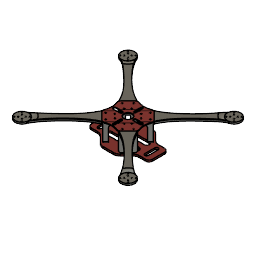
F450 Frame_GIT (Autodesk Fusion 360 design; units mm, degrees)
part number: 2026-06-03-11-10-49-567
Autodesk Fusion 360 part; units mm, degrees
sketch "Sketch1" plane through (0, 0, 0) normal (0, 0, 1) x (1, 0, 0)
  line L0 (-54, 54) -> (54, 54) construction
  line L1 (54, 54) -> (54, -54) construction
  line L2 (54, -54) -> (-54, -54) construction
  line L3 (-54, -54) -> (-54, 54) construction
  line L4 (-54, 54) -> (54, -54) construction
  line L5 (54, 54) -> (-54, -54) construction
  line L6 (-54, 24) -> (-24, 54)
  line L7 (24, 54) -> (54, 24)
  line L8 (54, -24) -> (24, -54)
  line L9 (-24, -54) -> (-54, -24)
  spline S0 degree 5 poles (-24, 54) (-23.04, 53.5449) (-21.12, 52.6745) (-18.24, 51.4881) (-14.4, 50.1486) (-9.6, 48.9056) (-4.8, 48.1327) (0, 47.868) (4.8, 48.1327) (9.6, 48.9056) (14.4, 50.1486) (18.24, 51.4881) (21.12, 52.6745) (23.04, 53.5449) (24, 54) knots 0 0 0 0 0 0 0.1 0.2 0.3 0.4 0.5 0.6 0.7 0.8 0.9 1 1 1 1 1 1
  spline S1 degree 5 poles (54, 24) (53.5449, 23.04) (52.6745, 21.12) (51.4881, 18.24) (50.1486, 14.4) (48.9056, 9.6) (48.1327, 4.8) (47.868, 0) (48.1327, -4.8) (48.9056, -9.6) (50.1486, -14.4) (51.4881, -18.24) (52.6745, -21.12) (53.5449, -23.04) (54, -24) knots 0 0 0 0 0 0 0.1 0.2 0.3 0.4 0.5 0.6 0.7 0.8 0.9 1 1 1 1 1 1
  spline S2 degree 5 poles (-24, -54) (-23.04, -53.5449) (-21.12, -52.6745) (-18.24, -51.4881) (-14.4, -50.1486) (-9.6, -48.9056) (-4.8, -48.1327) (0, -47.868) (4.8, -48.1327) (9.6, -48.9056) (14.4, -50.1486) (18.24, -51.4881) (21.12, -52.6745) (23.04, -53.5449) (24, -54) knots 0 0 0 0 0 0 0.1 0.2 0.3 0.4 0.5 0.6 0.7 0.8 0.9 1 1 1 1 1 1
  spline S3 degree 5 poles (-54, 24) (-53.5449, 23.04) (-52.6745, 21.12) (-51.4881, 18.24) (-50.1486, 14.4) (-48.9056, 9.6) (-48.1327, 4.8) (-47.868, 0) (-48.1327, -4.8) (-48.9056, -9.6) (-50.1486, -14.4) (-51.4881, -18.24) (-52.6745, -21.12) (-53.5449, -23.04) (-54, -24) knots 0 0 0 0 0 0 0.1 0.2 0.3 0.4 0.5 0.6 0.7 0.8 0.9 1 1 1 1 1 1
  circle A0 centre (-41.8284, 24.8579) radius 1.6
  circle A1 centre (-25.1436, 13.8299) radius 1.6
  circle A2 centre (-24.8579, 41.8284) radius 1.6
  circle A3 centre (-13.8299, 25.1436) radius 1.6
  line L10 (110, 0) -> (-135, 0) construction
  circle A4 centre (-13.8299, -25.1436) radius 1.6
  circle A5 centre (-25.1436, -13.8299) radius 1.6
  circle A6 centre (-41.8284, -24.8579) radius 1.6
  circle A7 centre (-24.8579, -41.8284) radius 1.6
  line L11 (0, 80) -> (0, -85.6972) construction
  circle A8 centre (41.8284, 24.8579) radius 1.6
  circle A9 centre (24.8579, 41.8284) radius 1.6
  circle A10 centre (13.8299, 25.1436) radius 1.6
  circle A11 centre (25.1436, 13.8299) radius 1.6
  circle A12 centre (25.1436, -13.8299) radius 1.6
  circle A13 centre (13.8299, -25.1436) radius 1.6
  circle A14 centre (24.8579, -41.8284) radius 1.6
  circle A15 centre (41.8284, -24.8579) radius 1.6
  point P0 (0, 48)
  point P1 (48, 0)
  point P2 (0, -48)
  point P3 (-48, 0)
  dimension "d1" = 108
  dimension "d2" = 108
  dimension "d3" = 30
  dimension "d4" = 30
  dimension "d5" = 30
  dimension "d6" = 45
  dimension "d7" = 30
  dimension "d8" = 45
  dimension "d9" = 6
  dimension "d10" = 6
  dimension "d11" = 6
  dimension "d12" = 6
  dimension "d13" = 3.2
  dimension "d14" = 3.2
  dimension "d15" = 8
  dimension "d16" = 12
  dimension "d17" = 8
  dimension "d18" = 20
  constraint horizontal L0
  constraint perpendicular L0 L1
  constraint parallel L0 L2
  constraint parallel L1 L3
  constraint coincident L4 origin
  constraint coincident L5 origin
  constraint coincident L3 L6.start
  constraint coincident L0 L6.end
  constraint coincident L0 L7.start
  constraint coincident L1 L7.end
  constraint coincident L1 L8.start
  constraint coincident L2 L8.end
  constraint perpendicular L4 L8
  constraint coincident L2 L9.start
  constraint coincident L3 L9.end
  constraint perpendicular L5 L9
  constraint symmetric L4 A0 A2
  constraint symmetric L4 A1 A3
  constraint horizontal L10
  constraint symmetric A0 L10 A6
  constraint symmetric A1 L10 A5
  constraint symmetric A2 L10 A7
  constraint symmetric A3 L10 A4
  constraint perpendicular L0 L11
  constraint symmetric A0 L11 A8
  constraint symmetric A1 L11 A11
  constraint symmetric A2 L11 A9
  constraint symmetric A3 L11 A10
  constraint symmetric A4 L11 A13
  constraint symmetric A5 L11 A12
  constraint symmetric A6 L11 A15
  constraint symmetric A7 L11 A14
  measures "d1" distance of L0.end L1.end
  measures "d2" distance of L0.start L0.end
  measures "d3" distance of L2.end L9.start
  measures "d4" distance of L1.end L8.end
  measures "d5" distance of L0.end L7.end
  measures "d6" angle of L0 L7
  measures "d7" distance of L0.start L6.end
  measures "d8" angle of L0 L6
  measures "d9" distance of L0 P0
  measures "d10" distance of L1 P1
  measures "d11" distance of L2 P2
  measures "d12" distance of L3 P3
  measures "d13" diameter of A0
  measures "d14" diameter of A1
  measures "d15" distance of L6 A0.centre
  measures "d16" distance of L4 A0.centre
  measures "d17" distance of L4 A1.centre
  measures "d18" distance of A0.centre A1.centre
extrude "Extrude1" add sketch "Sketch1" along normal blind 2 makes body 1
fillet "Fillet1" radius 10 8 edges at (-54, -24, 1) (-24, -54, 1) (24, -54, 1) (54, -24, 1) (-24, 54, 1) (-54, 24, 1) (24, 54, 1) (54, 24, 1) on bodies 1
sketch "Sketch2" plane through (0, 0, 2) normal (0, 0, 1) x (-1, 0, 0)
  spline S0 degree 3 poles (-49.2413, -28.7587) (-50.1621, -27.8379) (-50.8942, -26.7461) (-51.8987, -24.3434) (-52.1615, -23.0554) (-52.178, -20.5388) (-51.9647, -19.3329) (-51.5405, -18.1949) knots 0 0 0 0 0.390644 0.390644 0.781289 0.781289 1.145638 1.145638 1.145638 1.145638
  line L0 (-49.2413, -28.7587) -> (-28.7587, -49.2413)
  spline S1 degree 3 poles (-18.1949, -51.5405) (-19.4151, -51.9953) (-20.7124, -52.2074) (-23.3153, -52.1224) (-24.596, -51.8262) (-26.8918, -50.7953) (-27.8999, -50.1001) (-28.7587, -49.2413) knots 0 0 0 0 0.390644 0.390644 0.781289 0.781289 1.145638 1.145638 1.145638 1.145638
  spline S2 degree 5 poles (-18.1949, -51.5405) (-17.4359, -51.2576) (-15.717, -50.6459) (-13.038, -49.7969) (-9.399, -48.8733) (-4.8, -48.1327) (0, -47.868) (4.8, -48.1327) (9.399, -48.8733) (13.038, -49.7969) (15.717, -50.6459) (17.4359, -51.2576) (18.1949, -51.5405) knots -0.879061 -0.879061 -0.879061 -0.879061 -0.879061 -0.879061 -0.8 -0.7 -0.6 -0.5 -0.4 -0.3 -0.2 -0.120939 -0.120939 -0.120939 -0.120939 -0.120939 -0.120939
  spline S3 degree 3 poles (28.7587, -49.2413) (27.8379, -50.1621) (26.7461, -50.8942) (24.3434, -51.8987) (23.0554, -52.1615) (20.5388, -52.178) (19.3329, -51.9647) (18.1949, -51.5405) knots 0 0 0 0 0.390644 0.390644 0.781289 0.781289 1.145638 1.145638 1.145638 1.145638
  line L1 (28.7587, -49.2413) -> (49.2413, -28.7587)
  spline S4 degree 3 poles (51.5405, -18.1949) (51.9953, -19.4151) (52.2074, -20.7124) (52.1224, -23.3153) (51.8262, -24.596) (50.7953, -26.8918) (50.1001, -27.8999) (49.2413, -28.7587) knots 0 0 0 0 0.390644 0.390644 0.781289 0.781289 1.145638 1.145638 1.145638 1.145638
  spline S5 degree 5 poles (51.5405, -18.1949) (51.2576, -17.4359) (50.6459, -15.717) (49.7969, -13.038) (48.8733, -9.399) (48.1327, -4.8) (47.868, 0) (48.1327, 4.8) (48.8733, 9.399) (49.7969, 13.038) (50.6459, 15.717) (51.2576, 17.4359) (51.5405, 18.1949) knots 0.120939 0.120939 0.120939 0.120939 0.120939 0.120939 0.2 0.3 0.4 0.5 0.6 0.7 0.8 0.879061 0.879061 0.879061 0.879061 0.879061 0.879061
  spline S6 degree 3 poles (49.2413, 28.7587) (50.1621, 27.8379) (50.8942, 26.7461) (51.8987, 24.3434) (52.1615, 23.0554) (52.178, 20.5388) (51.9647, 19.3329) (51.5405, 18.1949) knots 0 0 0 0 0.390644 0.390644 0.781289 0.781289 1.145638 1.145638 1.145638 1.145638
  line L2 (49.2413, 28.7587) -> (28.7587, 49.2413)
  spline S7 degree 3 poles (18.1949, 51.5405) (19.4151, 51.9953) (20.7124, 52.2074) (23.3153, 52.1224) (24.596, 51.8262) (26.8918, 50.7953) (27.8999, 50.1001) (28.7587, 49.2413) knots 0 0 0 0 0.390644 0.390644 0.781289 0.781289 1.145638 1.145638 1.145638 1.145638
  spline S8 degree 5 poles (18.1949, 51.5405) (17.4359, 51.2576) (15.717, 50.6459) (13.038, 49.7969) (9.399, 48.8733) (4.8, 48.1327) (0, 47.868) (-4.8, 48.1327) (-9.399, 48.8733) (-13.038, 49.7969) (-15.717, 50.6459) (-17.4359, 51.2576) (-18.1949, 51.5405) knots 0.120939 0.120939 0.120939 0.120939 0.120939 0.120939 0.2 0.3 0.4 0.5 0.6 0.7 0.8 0.879061 0.879061 0.879061 0.879061 0.879061 0.879061
  spline S9 degree 3 poles (-28.7587, 49.2413) (-27.8379, 50.1621) (-26.7461, 50.8942) (-24.3434, 51.8987) (-23.0554, 52.1615) (-20.5388, 52.178) (-19.3329, 51.9647) (-18.1949, 51.5405) knots 0 0 0 0 0.390644 0.390644 0.781289 0.781289 1.145638 1.145638 1.145638 1.145638
  line L3 (-28.7587, 49.2413) -> (-49.2413, 28.7587)
  spline S10 degree 3 poles (-51.5405, 18.1949) (-51.9953, 19.4151) (-52.2074, 20.7124) (-52.1224, 23.3153) (-51.8262, 24.596) (-50.7953, 26.8918) (-50.1001, 27.8999) (-49.2413, 28.7587) knots 0 0 0 0 0.390644 0.390644 0.781289 0.781289 1.145638 1.145638 1.145638 1.145638
  spline S11 degree 5 poles (-51.5405, 18.1949) (-51.2576, 17.4359) (-50.6459, 15.717) (-49.7969, 13.038) (-48.8733, 9.399) (-48.1327, 4.8) (-47.868, 0) (-48.1327, -4.8) (-48.8733, -9.399) (-49.7969, -13.038) (-50.6459, -15.717) (-51.2576, -17.4359) (-51.5405, -18.1949) knots -0.879061 -0.879061 -0.879061 -0.879061 -0.879061 -0.879061 -0.8 -0.7 -0.6 -0.5 -0.4 -0.3 -0.2 -0.120939 -0.120939 -0.120939 -0.120939 -0.120939 -0.120939
  circle A0 centre (-24.8579, -41.8284) radius 1.6
  circle A1 centre (24.8579, -41.8284) radius 1.6
  circle A2 centre (-13.8299, -25.1436) radius 1.6
  circle A3 centre (25.1436, -13.8299) radius 1.6
  circle A4 centre (-13.8299, 25.1436) radius 1.6
  circle A5 centre (24.8579, 41.8284) radius 1.6
  circle A6 centre (41.8284, 24.8579) radius 1.6
  circle A7 centre (13.8299, -25.1436) radius 1.6
  circle A8 centre (-41.8284, -24.8579) radius 1.6
  circle A9 centre (41.8284, -24.8579) radius 1.6
  circle A10 centre (-41.8284, 24.8579) radius 1.6
  circle A11 centre (-24.8579, 41.8284) radius 1.6
  circle A12 centre (-25.1436, -13.8299) radius 1.6
  circle A13 centre (-25.1436, 13.8299) radius 1.6
  circle A14 centre (13.8299, 25.1436) radius 1.6
  circle A15 centre (25.1436, 13.8299) radius 1.6
  circle A16 centre (0, 0) radius 12.5
  line L4 (3, -42) -> (3, -20)
  arc A17 (3, -20) -> (-3, -20) centre (0, -20) ccw
  line L5 (-3, -20) -> (-3, -42)
  arc A18 (-3, -42) -> (3, -42) centre (0, -42) ccw
  line L6 (0, -42) -> (0, -20) construction
  line L7 (-20, 4) -> (-40, 4)
  arc A19 (-40, 4) -> (-40, -4) centre (-40, 0) ccw
  line L8 (-40, -4) -> (-20, -4)
  arc A20 (-20, -4) -> (-20, 4) centre (-20, 0) ccw
  line L9 (-20, 0) -> (-40, 0) construction
  line L10 (-77.8428, 0) -> (72.1572, 0) construction
  line L11 (0, -80) -> (0, 70) construction
  line L12 (40, -4) -> (20, -4)
  arc A21 (40, -4) -> (40, 4) centre (40, 0) ccw
  line L13 (20, 4) -> (40, 4)
  arc A22 (20, 4) -> (20, -4) centre (20, 0) ccw
  line L14 (-3, 20) -> (-3, 42)
  line L15 (3, 42) -> (3, 20)
  arc A23 (-3, 20) -> (3, 20) centre (0, 20) ccw
  arc A24 (3, 42) -> (-3, 42) centre (0, 42) ccw
  dimension "d23" = 25
  dimension "d24" = 6
  dimension "d25" = 8
  dimension "d26" = 20
  dimension "d27" = 150
  dimension "d28" = 150
  dimension "d29" = 20
  dimension "d30" = 20
  dimension "d31" = 22
  constraint coincident A16.centre origin
  constraint tangent L4 A17
  constraint tangent A17 L5
  constraint parallel L4 L5
  constraint tangent L5 A18
  constraint tangent L4 A18
  constraint vertical L6
  constraint tangent L7 A19
  constraint tangent A19 L8
  constraint parallel L7 L8
  constraint tangent L8 A20
  constraint tangent L7 A20
  constraint perpendicular L5 L9
  constraint horizontal L10
  constraint perpendicular L10 L11
  constraint collinear L9 L10
  constraint collinear L6 L11
  constraint symmetric L7.start L11 L13.start
  constraint symmetric L7.end L11 A21.end
  constraint symmetric A19.end L11 L12.start
  constraint symmetric L8.end L11 L12.end
  constraint symmetric A19 L11 A21
  constraint symmetric A20 L11 A22
  constraint symmetric L4.start L10 L15.start
  constraint symmetric L4.end L10 L15.end
  constraint symmetric A17.end L10 L14.start
  constraint symmetric L5.end L10 L14.end
  constraint symmetric A17 L10 A23
  constraint symmetric A18 L10 A24
  measures "d23" diameter of A16
  measures "d24" diameter of A17
  measures "d25" diameter of A19
  measures "d26" distance of A16.centre A20.centre
  measures "d27" distance of L10.start L10.end
  measures "d28" distance of L11.start L11.end
  measures "d29" distance of L7.start L7.end
  measures "d30" distance of A16.centre A17.centre
  measures "d31" distance of A17.end L5.end
extrude "Extrude2" cut sketch "Sketch2" against normal blind 2 contours A16 | L4 A17 L5 A18 | L7 A19 L8 A20 | L12 A21 L13 A22 | L14 L15 A23 A24 bodies 1
sketch "Sketch3" plane through (0, 0, 0) normal (0, 0, 1) x (1, 0, 0)
  line L0 (-65, 0) -> (70, 0) construction
  line L1 (0, -60) -> (0, 58.4085) construction
  line L2 (0, 0) -> (-176.7767, -176.7767) construction
  line L3 (-53.1421, -24.8579) -> (-24.8579, -53.1421)
  line L4 (-24.8579, -53.1421) -> (-6.4731, -34.7574)
  line L5 (-6.4731, -27.6863) -> (-27.6863, -6.4731)
  line L6 (-34.7574, -6.4731) -> (-53.1421, -24.8579)
  line L7 (-28.7587, -49.2413) -> (-49.2413, -28.7587)
  line L8 (-53.1421, -24.8579) -> (-171.9361, -143.6518) construction
  arc A0 (-27.6863, -6.4731) -> (-34.7574, -6.4731) centre (-31.2218, -10.0086) ccw
  arc A1 (-6.4731, -34.7574) -> (-6.4731, -27.6863) centre (-10.0086, -31.2218) ccw
  spline S0 degree 5 poles (-161.6105, -138.0992) (-160.6934, -137.7884) (-158.862, -137.1008) (-156.1235, -135.872) (-152.4419, -133.8154) (-147.5291, -130.4225) (-142.0023, -126.0691) (-135.6062, -120.6511) (-128.2424, -114.1593) (-120.0269, -106.7101) (-111.217, -98.5051) (-102.1675, -89.8068) (-93.2782, -80.9105) (-84.9455, -72.1182) (-77.5142, -63.7134) (-71.2254, -55.934) (-66.1683, -48.9471) (-62.2148, -42.8159) (-59.1194, -37.5347) (-56.6405, -33.0703) (-54.6445, -29.3984) (-53.5182, -27.1156) (-53.1237, -25.8179) (-53.0967, -25.1457) (-53.1421, -24.8579) knots 0 0 0 0 0 0 0.05 0.1 0.15 0.2 0.25 0.3 0.35 0.4 0.45 0.5 0.55 0.6 0.65 0.7 0.75 0.8 0.85 0.9 0.95 1 1 1 1 1 1
  line L9 (-51.7629, -33.5887) -> (-54.5214, -16.127)
  arc A2 (-162.4784, -138.3503) -> (-138.4805, -162.9894) centre (-157.7939, -157.7939) ccw
  spline S1 degree 5 poles (-137.3068, -160.2918) (-136.8023, -159.4836) (-135.7882, -157.8486) (-134.2519, -155.3405) (-132.1225, -151.8441) (-129.0449, -146.9999) (-125.2177, -141.4333) (-120.3455, -134.9473) (-114.2866, -127.4998) (-107.0974, -119.239) (-98.9687, -110.4365) (-90.1915, -101.4469) (-81.1134, -92.6595) (-72.101, -84.4542) (-63.5011, -77.1557) (-55.6013, -70.9864) (-48.5918, -66.0203) (-42.5198, -62.1251) (-37.3411, -59.0626) (-32.978, -56.603) (-29.3709, -54.6233) (-27.1046, -53.5111) (-25.8125, -53.123) (-25.1439, -53.0969) (-24.8579, -53.1421) knots 0 0 0 0 0 0 0.05 0.1 0.15 0.2 0.25 0.3 0.35 0.4 0.45 0.5 0.55 0.6 0.65 0.7 0.75 0.8 0.85 0.9 0.95 1 1 1 1 1 1
  line L10 (-33.5887, -51.7629) -> (-16.127, -54.5214)
  arc A3 (-162.4784, -138.3503) -> (-161.6105, -138.0992) centre (-164.8207, -128.6285) ccw
  arc A4 (-137.3068, -160.2918) -> (-138.4805, -162.9894) centre (-128.8238, -165.5871) ccw
  circle A5 centre (-169.3551, -169.3551) radius 1.6
  circle A6 centre (-163.3447, -163.3447) radius 1.6
  circle A7 centre (-152.2432, -163.3447) radius 1.6
  circle A8 centre (-146.2328, -169.3551) radius 1.6
  circle A9 centre (-152.2432, -152.2432) radius 1.6
  circle A10 centre (-146.2328, -146.2328) radius 1.6
  circle A11 centre (-163.3447, -152.2432) radius 1.6
  circle A12 centre (-169.3551, -146.2328) radius 1.6
  circle A13 centre (-41.8284, -24.8579) radius 1.6
  circle A14 centre (-25.1436, -13.8299) radius 1.6
  circle A15 centre (-13.8299, -25.1436) radius 1.6
  circle A16 centre (-24.8579, -41.8284) radius 1.6
  circle A17 centre (-41.8284, -24.8579) radius 2.5
  circle A18 centre (-24.8579, -41.8284) radius 2.5
  circle A19 centre (-13.8299, -25.1436) radius 2.5
  circle A20 centre (-25.1436, -13.8299) radius 2.5
  point P0 (-31.2218, -2.9376)
  point P1 (-137.4081, -122.1384)
  point P2 (-70.9005, -55.3064)
  point P3 (-55, -30)
  point P4 (-122.1384, -137.4081)
  point P5 (-55.3064, -70.9005)
  point P6 (-30, -55)
  dimension "d34" = 250
  dimension "d35" = 45
  dimension "d37" = 40
  dimension "d38" = 31
  dimension "d39" = 20
  dimension "d40" = 168
  dimension "d41" = 5
  dimension "d42" = 40
  dimension "d43" = 10
  dimension "d44" = 3.2
  dimension "d45" = 3.2
  dimension "d46" = 16.35
  dimension "d47" = 7.85
  dimension "d49" = 360
  dimension "d50" = 5
  dimension "d51" = 5
  dimension "d52" = 5
  dimension "d53" = 5
  constraint horizontal L0
  constraint perpendicular L0 L1
  constraint coincident L2.start origin
  constraint perpendicular L3 L4
  constraint parallel L3 L5
  constraint parallel L4 L6
  constraint perpendicular L2 L3
  constraint collinear L3 L7
  constraint parallel L2 L8
  constraint coincident P0 L5
  constraint coincident P0 L6
  constraint tangent L5 A0
  constraint tangent L6 A0
  constraint tangent L4 A1
  constraint tangent L5 A1
  constraint equal A0 A1
  constraint coincident L8.end A2
  constraint coincident L2 A2.centre
  constraint symmetric L2 L3.start L3.end
  constraint symmetric L2 P1 P4
  constraint symmetric L2 P2 P5
  constraint symmetric L2 P3 P6
  constraint midpoint L3.start L9
  constraint midpoint L3.end L10
  constraint tangent S0 A3
  constraint tangent A2 A3
  constraint tangent A2 A4
  constraint tangent S1 A4
  constraint equal A3 A4
  constraint coincident L2 A5.centre
  constraint coincident L2 A6.centre
  constraint concentric A13 A17
  constraint concentric A16 A18
  constraint concentric A15 A19
  constraint concentric A14 A20
  measures "d34" distance of L2.start L2.end
  measures "d35" angle of L1 L2
  measures "d37" distance of L3.start L3.end
  measures "d38" distance of L3.start P0
  measures "d39" distance of L2 L4
  measures "d40" distance of L3.start L8.end
  measures "d41" radius of A0
  measures "d42" diameter of A2
  measures "d43" radius of A3
  measures "d44" diameter of A5
  measures "d45" diameter of A6
  measures "d46" distance of A2.centre A5.centre
  measures "d47" distance of A2.centre A6.centre
  measures "d50" diameter of A17
  measures "d51" diameter of A18
  measures "d52" diameter of A19
  measures "d53" diameter of A20
extrude "Extrude3" add sketch "Sketch3" against normal blind 5 separate body contours L3 L4 L5 L6 L7 A0 A1 | L3 L7 S0 A2 S1 A3 A4 makes body 2
sketch "Sketch4" plane through (0, 0, -5) normal (0, 0, -1) x (1, 0, 0)
  circle A0 centre (-152.2432, 152.2432) radius 1.6
  circle A1 centre (-146.2328, 146.2328) radius 1.6
  line L0 (-6.4731, 34.7574) -> (-24.8579, 53.1421)
  spline S0 degree 5 poles (-24.8579, 53.1421) (-25.1439, 53.0969) (-25.8125, 53.123) (-27.1046, 53.5111) (-29.3709, 54.6233) (-32.978, 56.603) (-37.3411, 59.0626) (-42.5198, 62.1251) (-48.5918, 66.0203) (-55.6013, 70.9864) (-63.5011, 77.1557) (-72.101, 84.4542) (-81.1134, 92.6595) (-90.1915, 101.4469) (-98.9687, 110.4365) (-107.0974, 119.239) (-114.2866, 127.4998) (-120.3455, 134.9473) (-125.2177, 141.4333) (-129.0449, 146.9999) (-132.1225, 151.8441) (-134.2519, 155.3405) (-135.7882, 157.8486) (-136.8023, 159.4836) (-137.3068, 160.2918) knots -1 -1 -1 -1 -1 -1 -0.95 -0.9 -0.85 -0.8 -0.75 -0.7 -0.65 -0.6 -0.55 -0.5 -0.45 -0.4 -0.35 -0.3 -0.25 -0.2 -0.15 -0.1 -0.05 0 0 0 0 0 0
  arc A2 (-138.4805, 162.9894) -> (-137.3068, 160.2918) centre (-128.8238, 165.5871) ccw
  arc A3 (-138.4805, 162.9894) -> (-162.4784, 138.3503) centre (-157.7939, 157.7939) ccw
  arc A4 (-161.6105, 138.0992) -> (-162.4784, 138.3503) centre (-164.8207, 128.6285) ccw
  spline S1 degree 5 poles (-161.6105, 138.0992) (-160.6934, 137.7884) (-158.862, 137.1008) (-156.1235, 135.872) (-152.4419, 133.8154) (-147.5291, 130.4225) (-142.0023, 126.0691) (-135.6062, 120.6511) (-128.2424, 114.1593) (-120.0269, 106.7101) (-111.217, 98.5051) (-102.1675, 89.8068) (-93.2782, 80.9105) (-84.9455, 72.1182) (-77.5142, 63.7134) (-71.2254, 55.934) (-66.1683, 48.9471) (-62.2148, 42.8159) (-59.1194, 37.5347) (-56.6405, 33.0703) (-54.6445, 29.3984) (-53.5182, 27.1156) (-53.1237, 25.8179) (-53.0967, 25.1457) (-53.1421, 24.8579) knots 0 0 0 0 0 0 0.05 0.1 0.15 0.2 0.25 0.3 0.35 0.4 0.45 0.5 0.55 0.6 0.65 0.7 0.75 0.8 0.85 0.9 0.95 1 1 1 1 1 1
  line L1 (-53.1421, 24.8579) -> (-34.7574, 6.4731)
  arc A5 (-34.7574, 6.4731) -> (-27.6863, 6.4731) centre (-31.2218, 10.0086) ccw
  line L2 (-27.6863, 6.4731) -> (-6.4731, 27.6863)
  arc A6 (-6.4731, 27.6863) -> (-6.4731, 34.7574) centre (-10.0086, 31.2218) ccw
  circle A7 centre (-25.1436, 13.8299) radius 2.5
  circle A8 centre (-163.3447, 152.2432) radius 1.6
  circle A9 centre (-169.3551, 146.2328) radius 1.6
  circle A10 centre (-163.3447, 163.3447) radius 1.6
  circle A11 centre (-13.8299, 25.1436) radius 2.5
  circle A12 centre (-24.8579, 41.8284) radius 2.5
  circle A13 centre (-152.2432, 163.3447) radius 1.6
  circle A14 centre (-146.2328, 169.3551) radius 1.6
  circle A15 centre (-169.3551, 169.3551) radius 1.6
  circle A16 centre (-41.8284, 24.8579) radius 2.5
  line L3 (-43.2426, 14.9584) -> (-14.9584, 43.2426)
  line L4 (-23.4437, 51.7279) -> (-51.7279, 23.4437)
  dimension "d56" = 6
  dimension "d57" = 6
  constraint coincident L1 L3.start
  constraint coincident L0 L3.end
  constraint perpendicular L0 L3
  constraint coincident L0 L4.start
  constraint coincident L1 L4.end
  constraint parallel L3 L4
  measures "d56" distance of A12.centre L3
  measures "d57" distance of A12.centre L4
extrude "Extrude4" add sketch "Sketch4" along normal blind 50 contours L0 L1 L3 L4 bodies 2
sketch "Sketch5" plane through (-29.1005, -29.1005, 0) normal (0.707107, 0.707107, 0) x (-0.707107, 0.707107, 0)
  line L0 (20, -5) -> (-20, -5)
  line L1 (-20, -5) -> (-20, -55)
  line L2 (-20, -55) -> (20, -55)
  line L3 (20, -55) -> (20, -5)
  line L4 (7.5, -55) -> (4.5, -25)
  line L5 (4.5, -25) -> (-0.5, -25)
  line L6 (7.5, -55) -> (0, -55)
  line L7 (-0.1738, -70) -> (-0.1738, 16.5932) construction
  line L8 (-7.8476, -55) -> (-0.3476, -55)
  line L9 (-7.8476, -55) -> (-4.8476, -25)
  line L10 (-4.8476, -25) -> (0.1524, -25)
  dimension "d60" = 30
  dimension "d61" = 5
  dimension "d62" = 7.5
  constraint coincident L2 L4.start
  constraint parallel L2 L5
  constraint midpoint L2 L6.end
  constraint perpendicular L0 L7
  constraint symmetric L4.start L7 L8.start
  constraint symmetric L4.end L7 L9.end
  constraint symmetric L5.end L7 L10.end
  constraint symmetric L6.end L7 L8.end
  measures "d60" vertical distance of L4.start L4.end
  measures "d61" distance of L4.end L5.end
  measures "d62" distance of L4.start L6.end
extrude "Extrude5" cut sketch "Sketch5" against normal up to surface (12 mm away) contours L2 L4 L5 L6 L8 L9 L10 bodies 2
fillet "Fillet2" radius 1 4 edges at (-27.7941, -38.8922, -55) (-38.6464, -28.0398, -55) (-36.5251, -30.1612, -25) (-29.9154, -36.7709, -25) on bodies 2
fillet "Fillet2" radius 5 2 edges at (-19.201, -47.4853, -55) (-47.4853, -19.201, -55) on bodies 2
fillet "Fillet2" radius 10 1 edges at (-29.1005, -29.1005, -5) on bodies 2
fillet "Fillet2" radius 2 2 edges at (-24.8579, -53.1421, -2.5) (-53.1421, -24.8579, -2.5) on bodies 2
sketch "Sketch6" plane through (0, 0, 0) normal (0, 0, 1) x (-1, 0, 0)
  spline S0 degree 3 poles (53.1394, 25.4648) (53.1134, 25.2428) (53.0504, 25.0267) (52.8556, 24.6243) (52.7252, 24.4409) (52.5671, 24.2828) knots 0 0 0 0 0.067057 0.067057 0.134115 0.134115 0.134115 0.134115
  spline S1 degree 5 poles (161.6105, 138.0992) (160.6934, 137.7884) (158.862, 137.1008) (156.1235, 135.872) (152.4419, 133.8154) (147.5291, 130.4225) (142.0023, 126.0691) (135.6062, 120.6511) (128.2424, 114.1593) (120.0269, 106.7101) (111.217, 98.5051) (102.1675, 89.8068) (93.2782, 80.9105) (84.9455, 72.1182) (77.5142, 63.7134) (71.2254, 55.934) (66.1683, 48.9471) (62.2148, 42.8159) (59.1194, 37.5347) (56.6405, 33.0703) (54.7941, 29.6736) (53.7334, 27.5491) (53.2923, 26.3235) (53.1657, 25.6899) (53.1394, 25.4648) knots 0 0 0 0 0 0 0.05 0.1 0.15 0.2 0.25 0.3 0.35 0.4 0.45 0.5 0.55 0.6 0.65 0.7 0.75 0.8 0.85 0.9 0.95 0.981263 0.981263 0.981263 0.981263 0.981263 0.981263
  arc A0 (162.4784, 138.3503) -> (161.6105, 138.0992) centre (164.8207, 128.6285) ccw
  arc A1 (162.4784, 138.3503) -> (138.4805, 162.9894) centre (157.7939, 157.7939) ccw
  arc A2 (137.3068, 160.2918) -> (138.4805, 162.9894) centre (128.8238, 165.5871) ccw
  spline S2 degree 5 poles (137.3068, 160.2918) (136.8023, 159.4836) (135.7882, 157.8486) (134.2519, 155.3405) (132.1225, 151.8441) (129.0449, 146.9999) (125.2177, 141.4333) (120.3455, 134.9473) (114.2866, 127.4998) (107.0974, 119.239) (98.9687, 110.4365) (90.1915, 101.4469) (81.1134, 92.6595) (72.101, 84.4542) (63.5011, 77.1557) (55.6013, 70.9864) (48.5918, 66.0203) (42.5198, 62.1251) (37.3411, 59.0626) (32.978, 56.603) (29.6429, 54.7726) (27.5374, 53.725) (26.3189, 53.2901) (25.6889, 53.1653) (25.4656, 53.1393) knots 0 0 0 0 0 0 0.05 0.1 0.15 0.2 0.25 0.3 0.35 0.4 0.45 0.5 0.55 0.6 0.65 0.7 0.75 0.8 0.85 0.9 0.95 0.981146 0.981146 0.981146 0.981146 0.981146 0.981146
  spline S3 degree 3 poles (24.2826, 52.5669) (24.4408, 52.7251) (24.6244, 52.8556) (25.0271, 53.0505) (25.2434, 53.1134) (25.4656, 53.1393) knots 0 0 0 0 0.067109 0.067109 0.134217 0.134217 0.134217 0.134217
  line L0 (24.2826, 52.5669) -> (6.4731, 34.7574)
  arc A3 (6.4731, 34.7574) -> (6.4731, 27.6863) centre (10.0086, 31.2218) ccw
  line L1 (6.4731, 27.6863) -> (27.6863, 6.4731)
  arc A4 (27.6863, 6.4731) -> (34.7574, 6.4731) centre (31.2218, 10.0086) ccw
  line L2 (34.7574, 6.4731) -> (52.5671, 24.2828)
  circle A5 centre (152.2432, 152.2432) radius 1.6
  circle A6 centre (146.2328, 146.2328) radius 1.6
  circle A7 centre (25.1436, 13.8299) radius 2.5
  circle A8 centre (163.3447, 152.2432) radius 1.6
  circle A9 centre (169.3551, 146.2328) radius 1.6
  circle A10 centre (163.3447, 163.3447) radius 1.6
  circle A11 centre (13.8299, 25.1436) radius 2.5
  circle A12 centre (24.8579, 41.8284) radius 2.5
  circle A13 centre (152.2432, 163.3447) radius 1.6
  circle A14 centre (146.2328, 169.3551) radius 1.6
  circle A15 centre (169.3551, 169.3551) radius 1.6
  circle A16 centre (41.8284, 24.8579) radius 2.5
  line L3 (49.2413, 28.7587) -> (28.7587, 49.2413)
  spline S4 degree 3 poles (18.1949, 51.5405) (19.4151, 51.9953) (20.7124, 52.2074) (23.3153, 52.1224) (24.596, 51.8262) (26.8918, 50.7953) (27.8999, 50.1001) (28.7587, 49.2413) knots 0 0 0 0 0.390644 0.390644 0.781289 0.781289 1.145638 1.145638 1.145638 1.145638
  spline S5 degree 3 poles (49.2413, 28.7587) (50.1621, 27.8379) (50.8942, 26.7461) (51.8987, 24.3434) (52.1615, 23.0554) (52.178, 20.5388) (51.9647, 19.3329) (51.5405, 18.1949) knots 0 0 0 0 0.390644 0.390644 0.781289 0.781289 1.145638 1.145638 1.145638 1.145638
  circle A17 centre (157.7939, 157.7939) radius 20
  dimension "d73" = 40
  constraint concentric A1 A17
  measures "d73" diameter of A17
extrude "Extrude6" add sketch "Sketch6" along normal blind 2 separate body contours S0 S1 A0 A2 S2 S3 L0 L2 L3 S4 S5 A17 makes body 3
fillet "Fillet3" radius 50 1 edges at (-143.4666, -143.8395, 2) on bodies 3
mirror "Mirror1" about plane through (0, 0, 0) normal (0, 1, 0) of bodies 2 3 makes body 4 at (-119.5047, 114.7585, -5) makes body 5 at (-78.6021, 74.0861, 2)
mirror "Mirror2" about plane through (0, 0, 0) normal (1, 0, 0) of bodies 2 3 4 5 makes body 6 at (119.5047, -114.7585, -5) makes body 7 at (78.6021, -74.0861, 2) makes body 8 at (119.5047, 114.7585, -5) makes body 9 at (78.6021, 74.0861, 2)
sketch "Sketch7" plane through (0, 0, -55) normal (0, 0, -1) x (1, 0, 0)
  line L0 (18.4939, -39.7071) -> (26.9792, -48.1924)
  line L1 (26.9792, -48.1924) -> (31.3968, -43.7748)
  line L2 (31.3968, -43.7748) -> (22.9115, -35.2895)
  line L3 (22.9115, -35.2895) -> (18.4939, -39.7071)
  circle A0 centre (24.8579, -41.8284) radius 2.5
  line L4 (91, 59) -> (-91, 59) construction
  line L5 (-91, 59) -> (-91, -59) construction
  line L6 (-91, -59) -> (91, -59) construction
  line L7 (91, -59) -> (91, 59) construction
  line L8 (91, 59) -> (-91, -59) construction
  line L9 (-91, 59) -> (91, -59) construction
  line L10 (91, 0) -> (91, -18.5)
  line L11 (81, -28.5) -> (62.2843, -28.5)
  line L12 (48.1421, -34.3579) -> (29.3579, -53.1421)
  line L13 (0, -59) -> (15.2157, -59)
  line L14 (0, -100) -> (0, 90) construction
  line L15 (-150, 0) -> (150, 0) construction
  line L16 (0, -59) -> (-15.2157, -59)
  line L17 (-48.1421, -34.3579) -> (-29.3579, -53.1421)
  line L18 (-81, -28.5) -> (-62.2843, -28.5)
  line L19 (-91, 0) -> (-91, -18.5)
  line L20 (0, 59) -> (15.2157, 59)
  line L21 (0, 59) -> (-15.2157, 59)
  line L22 (-48.1421, 34.3579) -> (-29.3579, 53.1421)
  line L23 (48.1421, 34.3579) -> (29.3579, 53.1421)
  line L24 (81, 28.5) -> (62.2843, 28.5)
  line L25 (91, 0) -> (91, 18.5)
  line L26 (-81, 28.5) -> (-62.2843, 28.5)
  line L27 (-91, 0) -> (-91, 18.5)
  arc A1 (62.2843, -28.5) -> (48.1421, -34.3579) centre (62.2843, -48.5) ccw
  arc A2 (15.2157, -59) -> (29.3579, -53.1421) centre (15.2157, -39) ccw
  arc A3 (-29.3579, -53.1421) -> (-15.2157, -59) centre (-15.2157, -39) ccw
  arc A4 (-48.1421, -34.3579) -> (-62.2843, -28.5) centre (-62.2843, -48.5) ccw
  arc A5 (-62.2843, 28.5) -> (-48.1421, 34.3579) centre (-62.2843, 48.5) ccw
  arc A6 (-15.2157, 59) -> (-29.3579, 53.1421) centre (-15.2157, 39) ccw
  arc A7 (29.3579, 53.1421) -> (15.2157, 59) centre (15.2157, 39) ccw
  arc A8 (48.1421, 34.3579) -> (62.2843, 28.5) centre (62.2843, 48.5) ccw
  arc A9 (81, -28.5) -> (91, -18.5) centre (81, -18.5) ccw
  arc A10 (91, 18.5) -> (81, 28.5) centre (81, 18.5) ccw
  arc A11 (-81, 28.5) -> (-91, 18.5) centre (-81, 18.5) ccw
  arc A12 (-91, -18.5) -> (-81, -28.5) centre (-81, -18.5) ccw
  line L28 (41, -7.5) -> (-41, -7.5)
  arc A13 (-41, -7.5) -> (-41, -22.5) centre (-41, -15) ccw
  line L29 (-41, -22.5) -> (41, -22.5)
  arc A14 (41, -22.5) -> (41, -7.5) centre (41, -15) ccw
  line L30 (41, -15) -> (-41, -15) construction
  line L31 (-65, -15) -> (-65, 15)
  arc A15 (-65, 15) -> (-75, 15) centre (-70, 15) ccw
  line L32 (-75, 15) -> (-75, -15)
  arc A16 (-75, -15) -> (-65, -15) centre (-70, -15) ccw
  line L33 (-70, -15) -> (-70, 15) construction
  line L34 (41, 7.5) -> (-41, 7.5)
  line L35 (-41, 22.5) -> (41, 22.5)
  arc A17 (-41, 22.5) -> (-41, 7.5) centre (-41, 15) ccw
  arc A18 (41, 7.5) -> (41, 22.5) centre (41, 15) ccw
  arc A19 (65, -15) -> (75, -15) centre (70, -15) ccw
  line L36 (75, 15) -> (75, -15)
  line L37 (65, -15) -> (65, 15)
  arc A20 (75, 15) -> (65, 15) centre (70, 15) ccw
  point P0 (91, -28.5)
  point P1 (23.5, -59)
  dimension "d82" = 118
  dimension "d83" = 182
  dimension "d84" = 28.5
  dimension "d86" = 23.5
  dimension "d87" = 135
  dimension "d88" = 20
  dimension "d89" = 10
  dimension "d90" = 82
  dimension "d91" = 15
  dimension "d92" = 41
  dimension "d93" = 15
  dimension "d94" = 10
  dimension "d95" = 15
  constraint horizontal L4
  constraint perpendicular L4 L5
  constraint parallel L4 L6
  constraint parallel L5 L7
  constraint coincident L8 origin
  constraint coincident L9 origin
  constraint midpoint L7 L10.start
  constraint coincident L7 P0
  constraint perpendicular L10 L11
  constraint coincident L6 P1
  constraint midpoint L6 L13.start
  constraint vertical L14
  constraint perpendicular L7 L15
  constraint symmetric L10.start L14 L19.start
  constraint symmetric L13.start L14 L16.start
  constraint symmetric L10.start L15 L25.start
  constraint symmetric L13.start L15 L20.start
  constraint symmetric L15 L13.start L20.start
  constraint symmetric L15 L19.start L27.start
  constraint tangent L11 A1
  constraint tangent L12 A1
  constraint coincident P1 L12
  constraint coincident P1 L13
  constraint tangent L12 A2
  constraint tangent L13 A2
  constraint equal A1 A2
  constraint tangent L16 A3
  constraint tangent L17 A3
  constraint equal A1 A3
  constraint tangent L17 A4
  constraint tangent L18 A4
  constraint equal A1 A4
  constraint tangent L22 A5
  constraint tangent L26 A5
  constraint equal A1 A5
  constraint tangent L21 A6
  constraint tangent L22 A6
  constraint equal A1 A6
  constraint tangent L20 A7
  constraint tangent L23 A7
  constraint equal A1 A7
  constraint tangent L23 A8
  constraint tangent L24 A8
  constraint equal A1 A8
  constraint coincident P0 L10
  constraint coincident P0 L11
  constraint tangent L10 A9
  constraint tangent L11 A9
  constraint tangent L24 A10
  constraint tangent L25 A10
  constraint equal A9 A10
  constraint tangent L26 A11
  constraint tangent L27 A11
  constraint equal A9 A11
  constraint tangent L18 A12
  constraint tangent L19 A12
  constraint equal A9 A12
  constraint tangent L28 A13
  constraint tangent A13 L29
  constraint parallel L28 L29
  constraint tangent L29 A14
  constraint tangent L28 A14
  constraint parallel L15 L30
  constraint tangent L31 A15
  constraint tangent A15 L32
  constraint parallel L31 L32
  constraint tangent L32 A16
  constraint tangent L31 A16
  constraint perpendicular L15 L33
  constraint symmetric L15 L28.start L34.start
  constraint symmetric L15 L28.end L34.end
  constraint symmetric L15 A13.end L35.start
  constraint symmetric L15 L29.end L35.end
  constraint symmetric L15 A13 A17
  constraint symmetric L15 A14 A18
  constraint symmetric L14 L31.start A19.start
  constraint symmetric L14 L31.end L37.end
  constraint symmetric L14 A15.end L36.start
  constraint symmetric L14 L32.end A19.end
  constraint symmetric L14 A15 A20
  constraint symmetric L14 A16 A19
  measures "d82" distance of L4.end L5.end
  measures "d83" distance of L4.start L4.end
  measures "d84" distance of L10.start P0
  measures "d86" distance of P1 L13.start
  measures "d87" angle of L11 L12
  measures "d88" radius of A1
  measures "d89" radius of A9
  measures "d90" distance of A14.centre A13.centre
  measures "d91" diameter of A13
  measures "d92" distance of L14 A14.centre
  measures "d93" distance of L15 L30
  measures "d94" diameter of A15
  measures "d95" distance of L15 A15.centre
extrude "Extrude7" add sketch "Sketch7" along normal blind 5 separate body contours L0 L1 L2 L3 | A0 | L10 L11 L12 L13 L16 L17 L18 L19 L20 L21 L22 L23 L24 L25 L26 L27 A1 A2 A3 A4 A5 A6 A7 A8 A9 A10 A11 A12 makes body 10
named bodies: "Top", "Arm", "Arm Top", "Arm  (1)", "Arm Top (1)", "Arm  (2)", "Arm Top (2)", "Arm  (1) (1)", "Arm Top (1) (1)", "Base"
